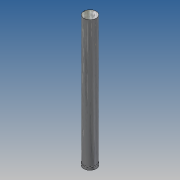
# Autodesk Inventor part: Axle
Saved by Autodesk Inventor 2015 (Build 190159000, 159)
## iProperties
Created: 2016-12-08
Part Number: Axle
Material: Allgemein
Document SubType Name: Modeling
Designer: NS
Density: 1 g/cm^3
Appearance: Aluminum - Dark
RuleStatus: InUse
BeforeDocSave0: file://C:\_Vault_ausgecheckt\ilogic\ipt
Author: NS
Autodesk Inventor part; units mm, degrees
ref_plane "YZ Plane" through (0, 0, 0) normal (1, 0, 0) x (0, 1, 0)
ref_plane "XZ Plane" through (0, 0, 0) normal (0, 1, 0) x (-1, 0, 0)
ref_plane "XY Plane" through (0, 0, 0) normal (0, 0, 1) x (1, 0, 0)
sketch "Sketch1" plane through (0, 0, 0) normal (0, 0, 1) x (1, 0, 0)
  circle A0 centre (0, 0) radius 2
  dimension "d0" = 4
  constraints: 1 centre point, 1 coincident
  measures "d0" diameter of A0
extrude "Extrusion1" add sketch "Sketch1" along normal blind 42
sketch "Sketch2" plane through (0, 0, 0) normal (1, 0, 0) x (0, 1, 0)
  line L0 (2, 1) -> (1.5, 1)
  line L1 (1.5, 1) -> (1.5, 0.8)
  line L2 (1.5, 0.8) -> (2, 0.8)
  line L3 (2, 0.8) -> (2, 1)
  line L4 (2, 42) -> (-2, 42)
  line L5 (-2, 0) -> (2, 0)
  line L6 (0, 0) -> (0, -0.918423) construction
  dimension "d3" = 0.5
  dimension "d4" = 0.2
  dimension "d5" = 0.8
  dimension "d6" = 1.5
  constraints: 10 end point, 2 parallel, 1 horizontal, 1 perpendicular, 1 vertical
  measures "d3" distance of L0.start L0.end
  measures "d4" distance of L2.end L0.start
  measures "d5" distance from line of L6.start L2
  measures "d6" distance from line of L1 L6.start
revolve "Revolution1" cut sketch "Sketch2" angle 360 about axis through (0, 0, 0) along (0, 0, -1)
sketch "Sketch4" plane through (0, 0, 42) normal (0, 0, 1) x (1, 0, 0)
  line L0 (0, 0) -> (-2, 0) construction
  circle A0 centre (0, 0) radius 2
  line L1 (-2, -0.105152) -> (-1.85, -0.105152)
  line L2 (-1.85, -0.105152) -> (-1.85, 0.094848)
  line L3 (-1.85, 0.094848) -> (-2, 0.094848)
  line L4 (-2, 0.094848) -> (-2, -0.105152)
  dimension "d10" = 0.2
  dimension "d11" = 0.15
  constraints: 10 end point, 2 horizontal, 2 parallel, 1 horizontal alignment, 1 perpendicular, 1 point on line, 1 other
  measures "d10" distance of L3.end L1.start
  measures "d11" distance of L2.end L3.end
sketch "Sketch4 outline for Extrusion2" plane through (0, 0, 42) normal (0, 0, 1) x (1, 0, 0)
  line L0 (-2, 0.094848) -> (-2, 0)
  line L1 (-1.85, 0.094848) -> (-2, 0.094848)
  line L2 (-1.85, -0.105152) -> (-1.85, 0.094848)
  line L3 (-2, -0.105152) -> (-1.85, -0.105152)
  line L4 (-2, 0) -> (-2, -0.105152)
extrude "Extrusion2" cut sketch "Sketch4 outline for Extrusion2" against normal blind 3
body "Solid1"
